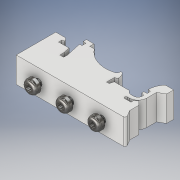
# Autodesk Inventor part: DINRailAdapter_PhoenixContact_1201578
Saved by Autodesk Inventor 2019.1 (Build 231200000, 200)
## iProperties
Created: 2018-10-29
Part Number: DINRailAdapter_PhoenixContact_1201578
Material: PC/ABS Plastic
Document SubType Name: Modeling
Designer: huesof
Density: 0.357273 g/cm^3
Appearance: Smooth - White
Mass: 1.98001 g
Surface Area: 28.826 cm^2
Volume: 5.54201 cm^3
Author: huesof
Autodesk Inventor part; units mm, degrees
ref_plane "YZ Plane" through (0, 0, 0) normal (1, 0, 0) x (0, 1, 0)
ref_plane "XZ Plane" through (0, 0, 0) normal (0, 1, 0) x (-1, 0, 0)
ref_plane "XY Plane" through (0, 0, 0) normal (0, 0, 1) x (1, 0, 0)
sketch "Sketch1" plane through (0, 0, 0) normal (0, 1, 0) x (-1, 0, 0)
  line L0 (0, 0) -> (21.245, 0)
  line L1 (0, 0) -> (-20.6799, 0)
  line L2 (-21.2644, -1.0125) -> (-19.895, -3.3844)
  line L3 (-21.849, 0) -> (-19.1101, 0) construction
  arc A0 (-20.6799, 0) -> (-21.2644, -1.0125) centre (-20.6799, -0.675) ccw
  line L4 (-19.895, -3.3844) -> (-19.895, -6.9494)
  line L5 (-19.895, -6.9494) -> (-18.415, -8.4294)
  line L6 (-19.895, -6.9494) -> (-17.802, -6.9494) construction
  line L7 (-18.415, -8.4294) -> (-17.295, -7.3093)
  line L8 (-17.295, -7.3093) -> (-17.295, -6.4493)
  line L9 (-17.295, -6.4493) -> (-14.828, -6.4493)
  line L10 (-14.303, -6.9743) -> (-14.303, -6.9743)
  line L11 (-14.828, -7.4993) -> (-15.608, -7.4993)
  arc A1 (-14.303, -6.9743) -> (-14.828, -6.4493) centre (-14.828, -6.9743) ccw
  arc A2 (-14.828, -7.4993) -> (-14.303, -6.9743) centre (-14.828, -6.9743) ccw
  arc A3 (-15.608, -7.4993) -> (-19.008, -10.8993) centre (-15.608, -10.8993) ccw
  line L12 (-15.608, -10.8993) -> (-19.008, -10.8993) construction
  line L13 (-15.608, -10.8993) -> (-15.608, -7.4993) construction
  line L14 (-19.008, -10.8993) -> (-19.008, -14.7753)
  line L15 (-19.008, -14.7753) -> (-21.5082, -16.2188)
  line L16 (-19.008, -14.7753) -> (-16.121, -14.7753) construction
  line L17 (-21.5082, -16.2188) -> (-21.5082, -19.0078)
  line L18 (-21.5082, -19.0078) -> (-18.2032, -19.0078)
  line L19 (-18.2032, -19.0078) -> (-16.4072, -19.0078) construction
  line L20 (-16.4072, -19.0078) -> (-16.4072, -14.1078) construction
  line L21 (-16.4072, -14.1078) -> (-17.4338, -13.9075)
  line L22 (-16.4072, -14.1078) -> (-15.3612, -14.1078) construction
  line L23 (-17.4338, -13.9075) -> (-17.5463, -12.5572)
  line L24 (-17.4338, -13.9075) -> (-16.0788, -13.9075) construction
  line L25 (-17.5463, -12.5572) -> (-16.2583, -12.5572)
  line L26 (-16.2583, -12.5572) -> (-16.2583, -11.8072)
  line L27 (-16.2583, -11.8072) -> (-17.5081, -11.2244)
  line L28 (-17.5081, -11.2244) -> (-17.5081, -10.7074)
  line L29 (-15.8081, -9.0074) -> (-14.8361, -9.0074)
  arc A4 (-15.8081, -9.0074) -> (-17.5081, -10.7074) centre (-15.8081, -10.7074) ccw
  line L30 (-14.8361, -9.0074) -> (-12.9081, -9.0074) construction
  line L31 (-12.9081, -9.0074) -> (-12.9081, -10.1074) construction
  line L32 (-12.9081, -10.1074) -> (-13.4221, -9.5934)
  line L33 (-12.9081, -10.1074) -> (-12.1811, -10.1074) construction
  line L34 (-12.9081, -10.1074) -> (-7.1081, -10.1074)
  line L35 (-7.1081, -10.1074) -> (-6.6795, -8.5079)
  line L36 (-7.1081, -10.1074) -> (-5.4521, -10.1074) construction
  line L37 (-6.6795, -8.5079) -> (-5.6835, -8.5079)
  line L38 (-5.6835, -8.5079) -> (-5.6835, -11.7279)
  line L39 (-5.6835, -11.7279) -> (-5.9885, -11.7279) construction
  line L40 (-5.9885, -11.7279) -> (-5.9885, -12.3579) construction
  arc A5 (-5.6835, -11.7279) -> (-6.6884, -12.3579) centre (-5.9885, -12.3579) ccw
  line L41 (-5.6835, -11.7279) -> (-5.2885, -11.7279) construction
  line L42 (-5.2885, -11.7279) -> (-5.2885, -14.4619) construction
  line L43 (-5.6835, -11.7279) -> (-3.3405, -11.7279) construction
  line L44 (-3.3405, -11.7279) -> (-3.3405, -12.2459) construction
  line L45 (-5.6835, -11.7279) -> (-5.5525, -11.7279) construction
  line L46 (-5.5525, -11.7279) -> (-5.5525, -14.7619) construction
  arc A6 (-5.5525, -14.7624) -> (-4.8885, -14.4619) centre (-5.2885, -14.4619) ccw
  line L47 (-5.6835, -11.7279) -> (7.9675, -11.7279) construction
  line L48 (7.9675, -11.7279) -> (7.9675, -17.3579) construction
  arc A7 (-3.6885, -13.2619) -> (-4.8885, -14.4619) centre (-3.6885, -14.4619) ccw
  line L49 (-3.6885, -14.4619) -> (-3.6885, -13.2619) construction
  line L50 (-3.6885, -14.4619) -> (-4.8885, -14.4619) construction
  arc A8 (7.9675, -17.3579) -> (-3.6885, -13.2619) centre (-0.878, -23.8967) ccw
  line L51 (7.9675, -17.3579) -> (9.7415, -17.3579)
  line L52 (9.7415, -17.3579) -> (9.7415, -19.0079)
  line L53 (9.7415, -19.0079) -> (12.6915, -19.0079)
  line L54 (12.6915, -19.0079) -> (12.6915, -17.7329)
  line L55 (12.6915, -17.7329) -> (11.5413, -17.6079)
  line L56 (11.5413, -17.6079) -> (11.5413, -16.1079)
  line L57 (11.5413, -16.1079) -> (12.3913, -16.1079)
  line L58 (12.3913, -16.1079) -> (12.3913, -15.6079)
  line L59 (12.3913, -15.6079) -> (11.1663, -10.0821)
  line L60 (11.1663, -10.0821) -> (11.1663, -8.5081)
  line L61 (11.1663, -8.5081) -> (12.6663, -8.5081)
  line L62 (12.6663, -8.5081) -> (12.6915, -10.3399)
  line L63 (12.6915, -10.3399) -> (13.2493, -12.7009)
  line L64 (13.2493, -12.7009) -> (17.3243, -12.7009)
  line L65 (17.3243, -12.7009) -> (17.3243, -13.9009)
  line L66 (17.3243, -13.9009) -> (16.5239, -14.1011)
  line L67 (16.5239, -14.1011) -> (16.5239, -14.5511)
  line L68 (16.5239, -14.5511) -> (17.4743, -15.5014)
  line L69 (17.4743, -15.5014) -> (21.245, -15.5014)
  line L70 (21.245, -15.5014) -> (21.245, 0)
  arc A9 (-18.2032, -19.0078) -> (-16.4072, -14.1078) centre (-23.8069, -14.1748) ccw
  arc A10 (-13.4221, -9.5934) -> (-14.8361, -9.0074) centre (-14.8365, -11.0074) ccw
  arc A11 (-6.6884, -12.3579) -> (-5.5525, -14.7624) centre (-3.3403, -12.2467) ccw
  point P0 (-14.303, -6.4493)
  point P1 (-14.303, -7.4993)
  point P2 (-17.5081, -9.0074)
  dimension "d0" = 21.245
  dimension "d1" = 21.849
  dimension "d2" = 3.908
  dimension "d3" = 60
  dimension "d4" = 0.675
  dimension "d5" = 3.565
  dimension "d6" = 45
  dimension "d7" = 2.093
  dimension "d8" = 1.584
  dimension "d9" = 0.86
  dimension "d10" = 2.992
  dimension "d11" = 1.05
  dimension "d12" = 1.305
  dimension "d13" = 0.525
  dimension "d14" = 90
  dimension "d15" = 3.4
  dimension "d16" = 3.876
  dimension "d17" = 2.887
  dimension "d18" = 150
  dimension "d19" = 2.789
  dimension "d20" = 3.305
  dimension "d21" = 1.796
  dimension "d22" = 4.9
  dimension "d25" = 1.046
  dimension "d26" = 168.96
  dimension "d27" = 265.24
  dimension "d28" = 1.355
  dimension "d29" = 1.288
  dimension "d30" = 0.75
  dimension "d31" = 1.379
  dimension "d32" = 115
  dimension "d33" = 2.217
  dimension "d35" = 2.672
  dimension "d36" = 1.7
  dimension "d37" = 1.928
  dimension "d38" = 1.1
  dimension "d39" = 0.727
  dimension "d40" = 135
  dimension "d41" = 5.8
  dimension "d44" = 1.656
  dimension "d45" = 75
  dimension "d46" = 0.996
  dimension "d47" = 3.22
  dimension "d48" = 0.305
  dimension "d49" = 0.63
  dimension "d50" = 0.395
  dimension "d51" = 2.734
  dimension "d52" = 2.343
  dimension "d53" = 0.518
  dimension "d54" = 0.131
  dimension "d55" = 3.034
  dimension "d57" = 0.4
  dimension "d58" = 13.651
  dimension "d59" = 5.63
  dimension "d60" = 90
  dimension "d61" = 1.2
  dimension "d62" = 0
  dimension "d63" = 11
  dimension "d64" = 1.774
  dimension "d65" = 1.65
  dimension "d66" = 2.95
  dimension "d67" = 1.275
  dimension "d68" = 1.157
  dimension "d69" = 96.2
  constraints: 142 end point, 25 perpendicular, 24 point on circle, 17 horizontal, 14 point on line, 12 centre point, 8 tangent, 7 equal length, 5 parallel, 4 vertical, 2 coincident, 1 concentric
  measures "d0" distance of L0.start L0.end
  measures "d1" distance of L0.start L3.start
  measures "d2" distance of L3.start L2.end
  measures "d3" angle of L2 L3
  measures "d4" radius of A0
  measures "d5" distance of L2.end L4.end
  measures "d6" angle of L5 L6
  measures "d7" distance of L4.end L5.end
  measures "d8" distance of L5.end L7.end
  measures "d9" distance of L7.end L8.end
  measures "d10" distance of L8.end point (-14.303, -6.449)
  measures "d11" distance of point (-14.303, -6.449) point (-14.303, -7.499)
  measures "d12" distance of point (-14.303, -7.499) L11.end
  measures "d13" radius of A1
  measures "d14" angle of L13 L12
  measures "d15" distance of L12.start L11.end
  measures "d16" distance of L12.end L14.end
  measures "d17" distance of L14.end L15.end
  measures "d18" angle of L15 L16
  measures "d19" distance of L15.end L17.end
  measures "d20" distance of L17.end L18.end
  measures "d21" distance of L18.end L19.end
  measures "d22" distance of L19.end L20.end
  measures "d25" distance of L20.end L21.end
  measures "d26" angle of L22 L21
  measures "d28" distance of L21.end L23.end
  measures "d29" distance of L23.end L25.end
  measures "d30" distance of L25.end L26.end
  measures "d31" distance of L26.end L27.end
  measures "d32" angle of L27 L26
  measures "d33" distance of L27.end point (-17.508, -9.007)
  measures "d35" distance of point (-17.508, -9.007) L29.end
  measures "d36" radius of A4
  measures "d37" distance of L29.end L30.end
  measures "d38" distance of L30.end L31.end
  measures "d39" distance of L31.end L32.end
  measures "d40" angle of L33 L32
  measures "d41" distance of L31.end L34.end
  measures "d44" distance of L34.end L35.end
  measures "d45" angle of L36 L35
  measures "d46" distance of L35.end L37.end
  measures "d47" distance of L37.end L38.end
  measures "d48" distance of L38.end L39.end
  measures "d49" distance of L39.end L40.end
  measures "d50" distance of L38.end L41.end
  measures "d51" distance of L41.end L42.end
  measures "d52" distance of L38.end L43.end
  measures "d53" distance of L43.end L44.end
  measures "d54" distance of L38.end L45.end
  measures "d55" distance of L45.end L46.end
  measures "d57" radius of A6
  measures "d58" distance of L38.end L47.end
  measures "d59" distance of L47.end L48.end
  measures "d60" angle of L49 L50
  measures "d61" distance of L50.end L49.start
  measures "d62" vertical distance of L42.end L50.end
  measures "d63" radius of A8
  measures "d64" distance of L48.end L51.end
  measures "d65" distance of L51.end L52.end
  measures "d66" distance of L52.end L53.end
  measures "d67" distance of L53.end L54.end
  measures "d68" distance of L54.end L55.end
  measures "d69" angle of L55 L54
extrude "Extrusion1" add sketch "Sketch1" along normal blind 5 and the other way blind 5
sketch "Sketch2" plane through (0, 0, 0) normal (0, 0, 1) x (1, 0, 0)
  point P0 (0, 0)
  point P1 (0, 0)
  point P2 (12.5, 0)
  point P3 (-12.5, 0)
  dimension "d95" = 12.5
  dimension "d96" = 12.5
  dimension "d97" = 0
  dimension "d98" = 0
  constraints: 1 coincident
  measures "d95" distance of point (0, 0) point (-12.5, 0)
  measures "d96" distance of point (12.5, 0) point (0, 0)
  measures "d97" vertical distance of point (0, 0) point (12.5, 0)
  measures "d98" vertical distance of point (-12.5, 0) point (0, 0)
hole "Hole1" at (0, 0, 0) at (12.5, 0, 0) at (-12.5, 0, 0) direction (0, 0, -1) diameter 2.75 depth 7.35
ref_plane "Work Plane1" through (-21.245, 5, 1.6) normal (0, 0, 1) x (1, 0, 0)
sketch "Sketch3" plane through (-21.245, 5, 1.6) normal (0, 0, 1) x (1, 0, 0)
  circle A0 centre (8.745, -5) radius 1.375 projected
  circle A1 centre (21.245, -5) radius 1.375 projected
  circle A2 centre (33.745, -5) radius 1.375 projected
  circle A3 centre (8.745, -5) radius 1.5
  circle A4 centre (21.245, -5) radius 1.5
  circle A5 centre (33.745, -5) radius 1.5
  circle A6 centre (8.745, -5) radius 2.575
  circle A7 centre (21.245, -5) radius 2.575
  circle A8 centre (33.745, -5) radius 2.575
  dimension "d107" = 3
  dimension "d108" = 3
  dimension "d109" = 3
  dimension "d118" = 5.15
  dimension "d119" = 5.15
  dimension "d120" = 5.15
  constraints: 6 centre point, 6 coincident
  measures "d107" diameter of A3
  measures "d108" diameter of A4
  measures "d109" diameter of A5
  measures "d118" diameter of A6
  measures "d119" diameter of A8
  measures "d120" diameter of A7
extrude "Extrusion2" add sketch "Sketch3" against normal blind 6 separate body contours A0 | A1 | A2
thread "Thread1" size "M3x0.5" class "6g" standard "ANSI Metric M Profile" full length
thread "Thread2" size "M3x0.5" class "6g" standard "ANSI Metric M Profile" full length
thread "Thread3" size "M3x0.5" class "6g" standard "ANSI Metric M Profile" full length
extrude "Extrusion3" add sketch "Sketch3" along normal blind 2.3 contours A0 | A1 | A2 | A3 | A4 | A5 | A6 | A7 | A8 bodies 2
fillet "Fillet1" radius 1.15 3 edges at (-15.075, 0, 3.9) (-2.575, 0, 3.9) (9.925, 0, 3.9)
ref_plane "Work Plane2" through (-21.245, 5, 3.9) normal (0, 0, 1) x (1, 0, 0)
sketch "Sketch5" plane through (-21.245, 5, 3.9) normal (0, 0, 1) x (1, 0, 0)
  circle A0 centre (21.245, -5) radius 0.9721 construction
  circle A1 centre (21.245, -5) radius 1.0751 construction
  circle A2 centre (21.245, -5) radius 1.3917 construction
  line L0 (0, 0) -> (41.9249, 0) construction
  line L1 (21.245, -5) -> (21.245, -4.0279) construction
  arc A3 (21.4769, -3.9502) -> (21.0131, -3.9502) centre (21.245, -4.0279) ccw
  line L2 (21.245, -5) -> (21.9409, -3.7948) construction
  line L3 (21.245, -5) -> (22.6367, -5) construction
  arc A4 (21.4769, -3.9502) -> (22.0382, -4.2742) centre (21.9409, -3.7948) ccw
  line L4 (21.245, -5) -> (21.245, -3.6083) construction
  line L5 (21.245, -5) -> (20.5492, -3.7948) construction
  line L6 (21.245, -5) -> (20.0398, -4.3041) construction
  line L7 (21.245, -5) -> (19.8533, -5) construction
  line L8 (21.245, -5) -> (20.0398, -5.6959) construction
  line L9 (21.245, -5) -> (20.5492, -6.2052) construction
  line L10 (21.245, -5) -> (21.245, -6.3917) construction
  line L11 (21.245, -5) -> (21.9409, -6.2052) construction
  line L12 (21.245, -5) -> (22.4502, -5.6959) construction
  line L13 (21.245, -5) -> (22.6367, -5) construction
  line L14 (21.245, -5) -> (22.4502, -4.3041) construction
  arc A5 (22.2701, -4.676) -> (22.0382, -4.2742) centre (22.0869, -4.5139) ccw
  arc A6 (22.2701, -4.676) -> (22.2701, -5.324) centre (22.6367, -5) ccw
  arc A7 (22.0382, -5.7258) -> (22.2701, -5.324) centre (22.0869, -5.4861) ccw
  arc A8 (22.0382, -5.7258) -> (21.4769, -6.0498) centre (21.9409, -6.2052) ccw
  arc A9 (21.0131, -6.0498) -> (21.4769, -6.0498) centre (21.245, -5.9721) ccw
  arc A10 (21.0131, -6.0498) -> (20.4518, -5.7258) centre (20.5492, -6.2052) ccw
  arc A11 (20.2199, -5.324) -> (20.4518, -5.7258) centre (20.4031, -5.4861) ccw
  arc A12 (20.2199, -5.324) -> (20.2199, -4.676) centre (19.8533, -5) ccw
  arc A13 (20.4518, -4.2742) -> (20.2199, -4.676) centre (20.4031, -4.5139) ccw
  arc A14 (20.4523, -4.2743) -> (21.0131, -3.9502) centre (20.5492, -3.7948) ccw
  line L15 (20.4523, -4.2743) -> (20.4518, -4.2742)
  circle A15 centre (8.745, -5) radius 1.425 projected
  arc A16 (32.7199, -5.324) -> (32.7199, -4.676) centre (32.3533, -5) ccw
  arc A17 (34.5382, -5.7258) -> (33.9769, -6.0498) centre (34.4409, -6.2052) ccw
  line L16 (33.745, -5) -> (34.4409, -6.2052) construction
  arc A18 (33.5131, -6.0498) -> (33.9769, -6.0498) centre (33.745, -5.9721) ccw
  line L17 (33.745, -5) -> (33.745, -6.3917) construction
  line L18 (33.745, -5) -> (32.5398, -5.6959) construction
  line L19 (33.745, -5) -> (33.0492, -6.2052) construction
  line L20 (33.745, -5) -> (32.3533, -5) construction
  line L21 (33.745, -5) -> (32.5398, -4.3041) construction
  line L22 (33.745, -5) -> (33.0492, -3.7948) construction
  line L23 (33.745, -5) -> (33.745, -4.0279) construction
  arc A19 (33.9769, -3.9502) -> (33.5131, -3.9502) centre (33.745, -4.0279) ccw
  line L24 (33.745, -5) -> (33.745, -3.6083) construction
  line L25 (33.745, -5) -> (34.4409, -3.7948) construction
  arc A20 (33.9769, -3.9502) -> (34.5382, -4.2742) centre (34.4409, -3.7948) ccw
  arc A21 (32.7199, -5.324) -> (32.9518, -5.7258) centre (32.9031, -5.4861) ccw
  arc A22 (32.9518, -4.2742) -> (32.7199, -4.676) centre (32.9031, -4.5139) ccw
  line L26 (32.9523, -4.2743) -> (32.9518, -4.2742)
  arc A23 (33.5131, -6.0498) -> (32.9518, -5.7258) centre (33.0492, -6.2052) ccw
  arc A24 (32.9523, -4.2743) -> (33.5131, -3.9502) centre (33.0492, -3.7948) ccw
  circle A25 centre (33.745, -5) radius 1.0751 construction
  circle A26 centre (33.745, -5) radius 1.3917 construction
  circle A27 centre (33.745, -5) radius 0.9721 construction
  line L27 (33.745, -5) -> (35.1367, -5) construction
  arc A28 (34.5382, -5.7258) -> (34.7701, -5.324) centre (34.5869, -5.4861) ccw
  line L28 (33.745, -5) -> (34.9502, -5.6959) construction
  arc A29 (34.7701, -4.676) -> (34.7701, -5.324) centre (35.1367, -5) ccw
  line L29 (33.745, -5) -> (35.1367, -5) construction
  line L30 (33.745, -5) -> (34.9502, -4.3041) construction
  arc A30 (34.7701, -4.676) -> (34.5382, -4.2742) centre (34.5869, -4.5139) ccw
  arc A31 (7.7199, -5.324) -> (7.7199, -4.676) centre (7.3533, -5) ccw
  arc A32 (9.5382, -5.7258) -> (8.9769, -6.0498) centre (9.4409, -6.2052) ccw
  line L31 (8.745, -5) -> (9.4409, -6.2052) construction
  arc A33 (8.5131, -6.0498) -> (8.9769, -6.0498) centre (8.745, -5.9721) ccw
  line L32 (8.745, -5) -> (8.745, -6.3917) construction
  line L33 (8.745, -5) -> (7.5398, -5.6959) construction
  line L34 (8.745, -5) -> (8.0492, -6.2052) construction
  line L35 (8.745, -5) -> (7.3533, -5) construction
  line L36 (8.745, -5) -> (7.5398, -4.3041) construction
  line L37 (8.745, -5) -> (8.0492, -3.7948) construction
  line L38 (8.745, -5) -> (8.745, -4.0279) construction
  arc A34 (8.9769, -3.9502) -> (8.5131, -3.9502) centre (8.745, -4.0279) ccw
  line L39 (8.745, -5) -> (8.745, -3.6083) construction
  line L40 (8.745, -5) -> (9.4409, -3.7948) construction
  arc A35 (8.9769, -3.9502) -> (9.5382, -4.2742) centre (9.4409, -3.7948) ccw
  arc A36 (7.7199, -5.324) -> (7.9518, -5.7258) centre (7.9031, -5.4861) ccw
  arc A37 (7.9518, -4.2742) -> (7.7199, -4.676) centre (7.9031, -4.5139) ccw
  line L41 (7.9523, -4.2743) -> (7.9518, -4.2742)
  arc A38 (8.5131, -6.0498) -> (7.9518, -5.7258) centre (8.0492, -6.2052) ccw
  arc A39 (7.9523, -4.2743) -> (8.5131, -3.9502) centre (8.0492, -3.7948) ccw
  circle A40 centre (8.745, -5) radius 1.0751 construction
  circle A41 centre (8.745, -5) radius 1.3917 construction
  circle A42 centre (8.745, -5) radius 0.9721 construction
  line L42 (8.745, -5) -> (10.1367, -5) construction
  arc A43 (9.5382, -5.7258) -> (9.7701, -5.324) centre (9.5869, -5.4861) ccw
  line L43 (8.745, -5) -> (9.9502, -5.6959) construction
  arc A44 (9.7701, -4.676) -> (9.7701, -5.324) centre (10.1367, -5) ccw
  line L44 (8.745, -5) -> (10.1367, -5) construction
  line L45 (8.745, -5) -> (9.9502, -4.3041) construction
  arc A45 (9.7701, -4.676) -> (9.5382, -4.2742) centre (9.5869, -4.5139) ccw
  arc A46 (20.2199, -5.324) -> (20.2199, -4.676) centre (19.8533, -5) ccw
  arc A47 (22.0382, -5.7258) -> (21.4769, -6.0498) centre (21.9409, -6.2052) ccw
  line L46 (21.245, -5) -> (21.9409, -6.2052) construction
  arc A48 (21.0131, -6.0498) -> (21.4769, -6.0498) centre (21.245, -5.9721) ccw
  line L47 (21.245, -5) -> (21.245, -6.3917) construction
  line L48 (21.245, -5) -> (20.0398, -5.6959) construction
  line L49 (21.245, -5) -> (20.5492, -6.2052) construction
  line L50 (21.245, -5) -> (19.8533, -5) construction
  line L51 (21.245, -5) -> (20.0398, -4.3041) construction
  line L52 (21.245, -5) -> (20.5492, -3.7948) construction
  line L53 (21.245, -5) -> (21.245, -4.0279) construction
  arc A49 (21.4769, -3.9502) -> (21.0131, -3.9502) centre (21.245, -4.0279) ccw
  line L54 (21.245, -5) -> (21.245, -3.6083) construction
  line L55 (21.245, -5) -> (21.9409, -3.7948) construction
  arc A50 (21.4769, -3.9502) -> (22.0382, -4.2742) centre (21.9409, -3.7948) ccw
  arc A51 (20.2199, -5.324) -> (20.4518, -5.7258) centre (20.4031, -5.4861) ccw
  arc A52 (20.4518, -4.2742) -> (20.2199, -4.676) centre (20.4031, -4.5139) ccw
  line L56 (20.4523, -4.2743) -> (20.4518, -4.2742)
  arc A53 (21.0131, -6.0498) -> (20.4518, -5.7258) centre (20.5492, -6.2052) ccw
  arc A54 (20.4523, -4.2743) -> (21.0131, -3.9502) centre (20.5492, -3.7948) ccw
  circle A55 centre (21.245, -5) radius 1.0751 construction
  circle A56 centre (21.245, -5) radius 1.3917 construction
  circle A57 centre (21.245, -5) radius 0.9721 construction
  line L57 (21.245, -5) -> (22.6367, -5) construction
  arc A58 (22.0382, -5.7258) -> (22.2701, -5.324) centre (22.0869, -5.4861) ccw
  line L58 (21.245, -5) -> (22.4502, -5.6959) construction
  arc A59 (22.2701, -4.676) -> (22.2701, -5.324) centre (22.6367, -5) ccw
  line L59 (21.245, -5) -> (22.6367, -5) construction
  line L60 (21.245, -5) -> (22.4502, -4.3041) construction
  arc A60 (22.2701, -4.676) -> (22.0382, -4.2742) centre (22.0869, -4.5139) ccw
  dimension "d151" = 2.1502
  dimension "d152" = 2.7834
  dimension "d150" = 1.9442
  dimension "d153" = 0.2446
  dimension "d154" = 60
  dimension "d157" = 360
  dimension "d161" = 12.5
  dimension "d164" = 12.5
  dimension "d167" = 12.5
  constraints: 120 end point, 120 point on circle, 52 centre point, 38 coincident, 20 point on line, 9 horizontal, 1 equal length, 1 perpendicular, 351 other
  measures "d150" diameter of A0
  measures "d153" radius of A3
  measures "d154" angle of L3 L2
  measures "d161" distance of point (21.245, -5) A15.centre
  measures "d164" distance of L6.end L21.end
  measures "d167" distance of L6.end L36.end
extrude "Extrusion4" cut sketch "Sketch5" against normal blind 1.3143 contours A4 A5 A6 A7 A8 A9 A10 A11 A12 A13 A14 A3 | A16 A22 A24 A19 A20 A30 A29 A28 A17 A18 A23 A21 | A31 A37 A39 A34 A35 A45 A44 A43 A32 A33 A38 A36 bodies 1 2
move or copy body "Move Body1" bodies to move or copy 1 2 copy no translate (0, 0, -1.6)
body "Solid1"
body "Solid2"
